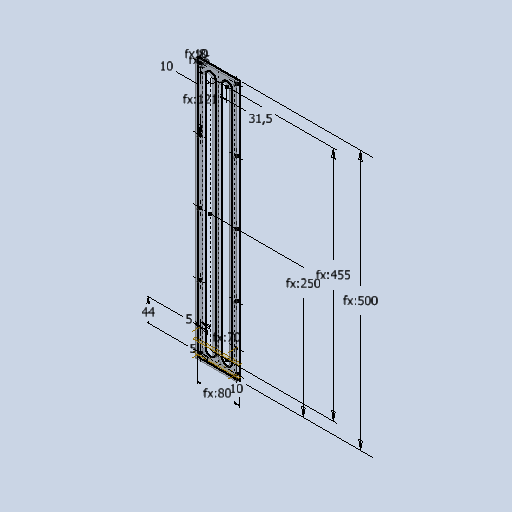
# Autodesk Inventor part: Slot profile
Saved by Autodesk Inventor 2022 (Build 260153000, 153)
## iProperties
Created: 2021-11-04
Part Number: Slot profile
Material: PMMA-Kunststoff
Document SubType Name: Modeling
Designer: espen
Density: 1.188 g/cm^3
Appearance: Polycarbonat - klar
Mass: 125.056 g
Surface Area: 583.529 cm^2
Volume: 105.266 cm^3
Author: espen
Autodesk Inventor part; units mm, degrees
ref_plane "YZ Plane" through (0, 0, 0) normal (1, 0, 0) x (0, 1, 0)
ref_plane "XZ Plane" through (0, 0, 0) normal (0, 1, 0) x (-1, 0, 0)
ref_plane "XY Plane" through (0, 0, 0) normal (0, 0, 1) x (1, 0, 0)
sketch "Sketch1" plane through (0, 0, 0) normal (0, 0, 1) x (1, 0, 0)
  line L0 (0, 0) -> (80, 0)
  line L1 (80, 0) -> (80, 500)
  line L2 (80, 500) -> (0, 500)
  line L3 (0, 500) -> (0, 0)
  line L4 (40, 500) -> (40, 0) construction
  line L5 (24.25, 477.5) -> (24.25, 22.5) construction
  line L6 (14.25, 477.5) -> (14.25, 22.5)
  line L7 (34.25, 22.5) -> (34.25, 477.5)
  arc A0 (34.25, 477.5) -> (14.25, 477.5) centre (24.25, 477.5) ccw
  arc A1 (14.25, 22.5) -> (34.25, 22.5) centre (24.25, 22.5) ccw
  circle A2 centre (5, 52) radius 2.5 construction
  circle A3 centre (5, 8) radius 2.5 construction
  line L8 (65.75, 477.5) -> (65.75, 22.5)
  line L9 (45.75, 22.5) -> (45.75, 477.5)
  arc A4 (65.75, 477.5) -> (45.75, 477.5) centre (55.75, 477.5) ccw
  arc A5 (45.75, 22.5) -> (65.75, 22.5) centre (55.75, 22.5) ccw
  circle A6 centre (75, 52) radius 2.5 construction
  circle A7 centre (75, 8) radius 2.5 construction
  circle A8 centre (5, 492) radius 1 construction
  circle A9 centre (75, 492) radius 1 construction
  line L10 (5, 8) -> (5, 52) construction
  circle A10 centre (5, 371) radius 1 construction
  circle A11 centre (75, 371) radius 1 construction
  circle A12 centre (5, 250) radius 1 construction
  circle A13 centre (75, 250) radius 1 construction
  circle A14 centre (5, 129) radius 1 construction
  circle A15 centre (75, 129) radius 1 construction
  circle A16 centre (5, 8) radius 1 construction
  circle A17 centre (75, 8) radius 1 construction
  line L11 (75, 8) -> (75, 52) construction
  line L12 (0, 500) -> (10, 500) construction
  line L13 (10, 500) -> (10, 0) construction
  line L14 (10, 0) -> (0, 0) construction
  line L15 (0, 0) -> (0, 500) construction
  line L16 (80, 500) -> (70, 500) construction
  line L17 (70, 500) -> (70, 0) construction
  line L18 (70, 0) -> (80, 0) construction
  line L19 (80, 0) -> (80, 500) construction
  line L20 (5, 8) -> (75, 8) construction
  line L21 (5, 8) -> (75, 8) construction
  point P0 (24.25, 250)
  dimension "d0" = 500
  dimension "d1" = 80
  dimension "d2" = 10
  dimension "d6" = 5
  dimension "d7" = 5
  dimension "d10" = 44
  dimension "d12" = 31.5
  dimension "d17" = 2
  dimension "d18" = 5
  dimension "d19" = 8
  dimension "d27" = 455
  dimension "d28" = 250
  dimension "d32" = 121
  dimension "d45" = 10
  dimension "d46" = 10
  dimension "d54" = 70
  constraints: 46 end point, 18 centre point, 14 coincident, 9 symmetric about line, 8 parallel, 8 point on circle, 5 perpendicular, 4 horizontal, 4 tangent, 3 midpoint, 3 vertical, 2 point on line, 1 collinear, 21 other
  measures "d0" distance of L0.end L1.end
  measures "d1" distance of L0.start L0.end
  measures "d2" radius of A0
  measures "d6" diameter of A2
  measures "d7" diameter of A3
  measures "d10" distance of L10.start L10.end
  measures "d12" distance of A4.centre L5.start
  measures "d17" diameter of A8
  measures "d18" distance from line of L3 A8.centre
  measures "d19" distance from line of A8.centre L2
  measures "d27" distance of L5.start L5.end
  measures "d28" distance from line of point (24.25, 250) L0
  measures "d32" distance of A8.centre A10.centre
  measures "d45" distance between parallel lines of L3 L13
  measures "d46" distance between parallel lines of L1 L17
  measures "d54" distance between parallel lines of L11 L10
extrude "Extrusion1" add sketch "Sketch1" along normal blind 5
hole "Bohrung1" at (5, 52, 0) at (5, 8, 0) at (75, 8, 0) at (75, 52, 0) direction (0, 0, 1) diameter 3.4 depth 11.8 tip angle 118 clearance for "Inbusschraube DIN EN ISO 4762" size "M3" standard "DIN"
hole "Bohrung2" at (5, 492, 0) at (75, 492, 0) at (5, 371, 0) at (75, 371, 0) at (5, 250, 0) at (75, 250, 0) at (5, 129, 0) at (75, 129, 0) at (5, 8, 0) at (75, 8, 0) direction (0, 0, 1) diameter 3.4 end through all clearance for "Inbusschraube DIN EN ISO 4762" size "M3" standard "DIN"
ref_plane "Arbeitsebene2" through (5, 30, 5.9) normal (0, 1, 0) x (0, 0, 1)
ref_plane "Arbeitsebene1" through (5, 8, 5.9) normal (0, 1, 0) x (0, 0, 1)
sketch "Skizze2" plane through (0, 0, 5) normal (0, 0, 1) x (1, 0, 0)
  line L0 (-16, 30) -> (96, 30) construction
  line L1 (40, 500) -> (40, 0) construction
  point P0 (0, 0)
  point P1 (40, 38)
  point P2 (40, 22)
  dimension "d56" = 8
  dimension "d57" = 8
  constraints: 2 point on line
  measures "d56" distance from line of L0 point (40, 22)
  measures "d57" distance from line of L0 point (40, 38)
hole "Bohrung3" at (40, 22, 5) at (40, 38, 5) direction (0, 0, -1) diameter 2.459 depth 8.8 tip angle 118 thread size "M3x0.5" class "6H" standard "ISO Metric profile"
equation "\"d0\" = GuidanceTrack_Length"
equation "\"d1\" = BackPlate_Width"
equation "\"d18\" = 0.5 * GuidanceTrac_OneSide_Thickness"
equation "\"d19\" = TopLit_Fixhole_Edge_Dist"
equation "\"d28\" = 0.5 * d0"
equation "\"d54\" = Guidacne_fixHoleDist"
equation "\"d57\" = d56"
equation "\"GuidanceTrack_Length\" = 500"
equation "\"BackPlate_Width\" = 80"
equation "\"GuidanceTrac_OneSide_Thickness\" = 10"
equation "\"TopLit_Fixhole_Edge_Dist\" = 8"
equation "\"Guidacne_fixHoleDist\" = 70"
body "Solid1"
